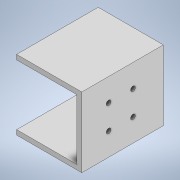
# Autodesk Inventor part: soporte 2.0
Saved by Autodesk Inventor 2020.3 (Build 243373000, 373)
## iProperties
Created: 2021-02-09
Part Number: soporte 2.0
Material: Generic
Document SubType Name: Modeling
Designer: Yu Jinyu
Density: 1 g/cm^3
Appearance: Default
Author: Yu Jinyu
Autodesk Inventor part; units mm, degrees
ref_plane "YZ Plane" through (0, 0, 0) normal (1, 0, 0) x (0, 1, 0)
ref_plane "XZ Plane" through (0, 0, 0) normal (0, 1, 0) x (-1, 0, 0)
ref_plane "XY Plane" through (0, 0, 0) normal (0, 0, 1) x (1, 0, 0)
sketch "Sketch1" plane through (0, 0, 0) normal (0, 0, 1) x (1, 0, 0)
  line L0 (-31.45, -31.45) -> (31.45, -31.45)
  line L1 (31.45, -31.45) -> (31.45, 31.45)
  line L2 (31.45, 31.45) -> (-31.45, 31.45)
  line L3 (-31.45, 31.45) -> (-31.45, -31.45)
  line L4 (-31.45, -31.45) -> (31.45, 31.45) construction
  line L5 (31.45, -31.45) -> (-31.45, 31.45) construction
  line L6 (-36.45, 36.45) -> (36.45, 36.45)
  line L7 (36.45, 36.45) -> (36.45, -36.45)
  line L8 (36.45, -36.45) -> (-36.45, -36.45)
  line L9 (-36.45, -36.45) -> (-36.45, 36.45)
  point P0 (0, 0)
  dimension "d0" = 62.9
  dimension "d1" = 62.9
  dimension "d2" = 5
  constraints: 20 end point, 4 parallel, 2 midpoint, 2 perpendicular, 1 horizontal, 3 other
  measures "d0" distance of L2.end L1.end
  measures "d1" distance of L1.end L0.end
  measures "d2" distance between parallel lines of L2 L6
extrude "Extrusion1" add sketch "Sketch1" along normal blind 85
sketch "Sketch2" plane through (0, 0, 0) normal (0, 0, -1) x (-1, 0, 0)
  line L0 (31.45, 31.45) -> (-31.45, 31.45) projected
  line L1 (31.45, -31.45) -> (-31.45, -31.45)
  line L2 (-31.45, -31.45) -> (-31.45, 31.45)
  line L3 (-31.45, 31.45) -> (31.45, 31.45)
  line L4 (31.45, 31.45) -> (31.45, -31.45)
  line L5 (31.45, -31.45) -> (-31.45, 31.45) construction
  line L6 (-31.45, -31.45) -> (31.45, 31.45) construction
  point P0 (0, 0)
  point P1 (31.45, 31.45)
  constraints: 12 end point, 2 midpoint, 2 parallel, 1 horizontal, 1 perpendicular
extrude "Extrusion2" add sketch "Sketch2" against normal blind 12.144
sketch "Sketch3" plane through (-36.45, -36.45, 0) normal (-1, 0, 0) x (0, 0, 1)
  line L0 (85, 0) -> (85, 72.9) projected
  line L1 (85, 0) -> (0, 0)
  line L2 (0, 0) -> (0, 67.9)
  line L3 (0, 67.9) -> (85, 67.9)
  line L4 (85, 67.9) -> (85, 0)
  point P0 (0, 36.45)
  constraints: 8 end point, 2 parallel, 1 horizontal, 1 perpendicular
extrude "Extrusion3" cut sketch "Sketch3" against normal blind 5
sketch "Sketch4" plane through (0, 0, 0) normal (0, 0, -1) x (-1, 0, 0)
  point P0 (0, 0)
sketch "Sketch5" plane through (-36.45, 31.45, 0) normal (-1, 0, 0) x (0, 0, 1)
  line L0 (0, 5) -> (0, 0) projected
  line L1 (0, 5) -> (85, 5) projected
  line L2 (0, 0) -> (85, 0) projected
  line L3 (85, 5) -> (85, 0) projected
  point P0 (0, -31.45)
extrude "Extrusion4" cut sketch "Sketch5" against normal blind 5
sketch "Sketch6" plane through (0, 0, 0) normal (0, 0, -1) x (-1, 0, 0)
  circle A0 centre (0, 0) radius 22.545
  dimension "d11" = 45.09
  constraints: 1 centre point, 1 coincident
  measures "d11" diameter of A0
extrude "Extrusion5" cut sketch "Sketch6" against normal blind 5
sketch "Sketch7" plane through (0, 0, 5) normal (0, 0, -1) x (-1, 0, 0)
  circle A0 centre (0, 0) radius 25.4
  dimension "d14" = 50.8
  constraints: 1 centre point, 1 coincident
  measures "d14" diameter of A0
sketch "Sketch8" plane through (0, 0, 12.144) normal (0, 0, 1) x (1, 0, 0)
  point P0 (0, 0)
extrude "Extrusion6" cut sketch "Sketch7" against normal blind 10
sketch "Sketch12" plane through (36.45, 36.45, 85) normal (0, 1, 0) x (1, 0, 0)
  circle A0 centre (-33.8267, 41.9258) radius 12.7 projected
  point P0 (-36.45, 85)
extrude "Extrusion10" cut sketch "Sketch12" along normal blind 5
sketch "Sketch13" plane through (31.45, -31.45, 85) normal (-1, 0, 0) x (0, 0, 1)
  ellipse E0 centre (-53.33, 18.7291) end of major axis (-50.83, 18.7291) minor radius 2.5 projected
  ellipse E1 centre (-27.93, 44.1291) end of major axis (-25.43, 44.1291) minor radius 2.5 projected
  ellipse E2 centre (-53.33, 44.1291) end of major axis (-50.83, 44.1291) minor radius 2.5 projected
  ellipse E3 centre (-27.93, 18.7291) end of major axis (-25.43, 18.7291) minor radius 2.5 projected
  point P0 (-85, 31.45)
extrude "Extrusion11" cut sketch "Sketch13" against normal blind 5
sketch "Sketch14" plane through (-31.45, -36.45, 0) normal (-1, 0, 0) x (0, 0, 1)
  circle A0 centre (6.072, 70.4) radius 1.5
  line L0 (0, 72.9) -> (85, 72.9) projected
  line L1 (0, 0) -> (0, 67.9) projected
  line L2 (12.144, 5) -> (12.144, 67.9) projected
  circle A1 centre (6.072, 2.5) radius 1.5
  line L3 (85, 0) -> (0, 0) projected
  circle A2 centre (78.928, 70.4) radius 1.5
  circle A3 centre (78.928, 2.5) radius 1.5
  line L4 (85, 5) -> (85, 0) projected
  point P0 (0, 36.45)
  dimension "d43" = 3
  dimension "d44" = 2.5
  dimension "d45" = 6.072
  dimension "d46" = 12.144
  dimension "d47" = 3
  dimension "d48" = 2.5
  dimension "d49" = 6.072
  dimension "d50" = 3
  dimension "d51" = 6.072
  dimension "d52" = 2.5
  dimension "d53" = 3
  dimension "d54" = 6.072
  constraints: 4 centre point
  measures "d43" diameter of A0
  measures "d44" distance from line of A0.centre L0
  measures "d45" distance from line of A0.centre L1
  measures "d46" distance between parallel lines of L2 L1
  measures "d47" diameter of A1
  measures "d48" distance from line of L3 A1.centre
  measures "d49" distance from line of A1.centre L1
  measures "d50" diameter of A2
  measures "d51" horizontal distance of L0.end A2.centre
  measures "d52" distance from line of L0 A2.centre
  measures "d53" diameter of A3
  measures "d54" distance from line of L4 A3.centre
extrude "Extrusion12" cut sketch "Sketch14" against normal blind 5
thread "Thread5" size "M3x0.5" class "6H" standard "ANSI Metric M Profile" full length
thread "Thread6" size "M3x0.5" class "6H" standard "ANSI Metric M Profile" full length
thread "Thread7" size "M3x0.5" class "6H" standard "ANSI Metric M Profile" full length
thread "Thread8" size "M3x0.5" class "6H" standard "ANSI Metric M Profile" full length
sketch "Sketch15" plane through (36.45, -36.45, 0) normal (0, -1, 0) x (1, 0, 0)
  circle A0 centre (-33.8267, 43.0742) radius 12.7 projected
  circle A1 centre (-33.8267, 43.0742) radius 4.775
  point P0 (-36.45, 0)
  dimension "d65" = 9.55
  constraints: 1 centre point, 1 coincident
  measures "d65" diameter of A1
extrude "Extrusion13" cut sketch "Sketch15" against normal blind 5 contours A1
body "Solid1"
